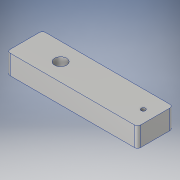
# Autodesk Inventor part: Transmisor_grande
Saved by Autodesk Inventor 2019 (Build 230136000, 136)
## iProperties
Created: 2019-09-30
Part Number: Transmisor_grande
Material: Aluminum 6061
Document SubType Name: Modeling
Designer: Domenico
Density: 2.7 g/cm^3
Appearance: Aluminum - Flat
Mass: 248.957 g
Surface Area: 184.654 cm^2
Volume: 92.2063 cm^3
Author: Domenico
Autodesk Inventor part; units mm, degrees
ref_plane "YZ Plane" through (0, 0, 0) normal (1, 0, 0) x (0, 1, 0)
ref_plane "XZ Plane" through (0, 0, 0) normal (0, 1, 0) x (-1, 0, 0)
ref_plane "XY Plane" through (0, 0, 0) normal (0, 0, 1) x (1, 0, 0)
sketch "Sketch1" plane through (0, 0, 0) normal (0, 1, 0) x (-1, 0, 0)
  line L0 (0, 0) -> (-120, 0)
  line L1 (-120, 0) -> (-120, -32.7)
  line L2 (-120, -32.7) -> (0, -32.7)
  line L3 (0, -32.7) -> (0, 0)
  circle A0 centre (-33, -16.35) radius 5.5563
  circle A1 centre (-108.8875, -16.35) radius 2
  point P0 (0, -16.35)
  point P1 (-120, -16.35)
  dimension "d0" = 120
  dimension "d1" = 32.7
  dimension "d2" = 33
  dimension "d3" = 11.1125
  dimension "d4" = 11.1125
  dimension "Diametro_eje_pequeño" = 4
  constraints: 8 end point, 2 centre point, 2 horizontal alignment, 2 midpoint, 2 parallel, 1 horizontal, 1 perpendicular
  measures "d0" distance of L2.end L1.end
  measures "d1" distance of L0.end L1.end
  measures "d2" distance from line of L3 A0.centre
  measures "d3" diameter of A0
  measures "d4" distance from line of L1 A1.centre
  measures "Diametro_eje_pequeño" diameter of A1
extrude "Extrusion1" add sketch "Sketch1" along normal blind 18
fillet "Fillet1" radius 3 4 edges at (0, 9, 0) (120, 9, 0) (120, 9, -32.7) (0, 9, -32.7)
equation "\"d1\" = ancho"
equation "\"d2\" = separacion_grande"
equation "\"d3\" = diametro_interno"
equation "\"d4\" = d3"
equation "\"Diametro_eje_pequeño\" = Diametro_eje_pequeño_1"
equation "\"ancho\" = 32.7"
equation "\"separacion_grande\" = 33"
equation "\"diametro_interno\" = 11.1125"
equation "\"Diametro_eje_pequeño_1\" = 4"
body "Solid1"
